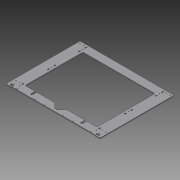
# Autodesk Inventor part: main_frame
Saved by Autodesk Inventor 2013 (Build 170138000, 138)
## iProperties
Created: 2013-11-17
Part Number: main_frame
Material: Generic
Document SubType Name: Modeling
Designer: Masta
Density: 1 g/cm^3
Author: Masta
Autodesk Inventor part; units mm, degrees
ref_plane "YZ Plane" through (0, 0, 0) normal (1, 0, 0) x (0, 1, 0)
ref_plane "XZ Plane" through (0, 0, 0) normal (0, 1, 0) x (-1, 0, 0)
ref_plane "XY Plane" through (0, 0, 0) normal (0, 0, 1) x (1, 0, 0)
sketch "Sketch1" plane through (0, 0, 0) normal (0, 0, 1) x (1, 0, 0)
  line L0 (36.0471, 18.5032) -> (31.0471, 23.3114)
  line L1 (31.0471, 383.5032) -> (36.0471, 388.5032)
  line L2 (36.0471, 388.5032) -> (396.0471, 388.5032)
  line L3 (396.0471, 388.5032) -> (401.0471, 383.5032)
  line L4 (401.0471, 23.5032) -> (396.0471, 18.5032)
  line L5 (376.0471, 18.5032) -> (374.0471, 20.5032)
  line L6 (374.0471, 20.5032) -> (58.0471, 20.5032)
  line L7 (58.0471, 20.5032) -> (56.0471, 18.5032)
  line L8 (111.0471, 58.5032) -> (91.0471, 58.5032)
  line L9 (91.0471, 58.5032) -> (86.0471, 63.5032)
  line L10 (86.0471, 63.5032) -> (86.0471, 343.5032)
  line L11 (86.0471, 343.5032) -> (91.0471, 348.5032)
  line L12 (91.0471, 348.5032) -> (341.0471, 348.5032)
  line L13 (341.0471, 348.5032) -> (346.0471, 343.5032)
  line L14 (346.0471, 343.5032) -> (346.0471, 63.5032)
  line L15 (346.0471, 63.5032) -> (341.0471, 58.5032)
  line L16 (341.0471, 58.5032) -> (321.0471, 58.5032)
  line L17 (211.0471, 33.5032) -> (221.0471, 33.5032)
  line L18 (221.0471, 33.5032) -> (246.0471, 58.5032)
  line L19 (211.0471, 33.5032) -> (186.0471, 58.5032)
  line L20 (141.0471, 58.5032) -> (186.0471, 58.5032)
  line L21 (246.0471, 58.5032) -> (291.0471, 58.5032)
  line L22 (381.0471, 24.5032) -> (381.3268, 24.54)
  line L23 (31.0471, 23.3114) -> (31.0471, 383.5032)
  line L24 (401.0471, 383.5032) -> (401.0471, 23.5032)
  line L25 (396.0471, 18.5032) -> (376.0471, 18.5032) construction
  line L26 (56.0471, 18.5032) -> (36.0471, 18.5032)
  line L27 (373.147, 30.54) -> (372.7474, 29.5753)
  line L28 (372.6111, 28.54) -> (372.7474, 27.5047)
  line L29 (375.5758, 32.4037) -> (374.6111, 32.0041)
  line L30 (385.6423, 32.4037) -> (384.6071, 32.54)
  line L31 (387.4355, 25.7116) -> (388.0712, 26.54)
  line L32 (386.6071, 25.0759) -> (387.4355, 25.7116)
  line L33 (385.6423, 24.6763) -> (386.6071, 25.0759)
  line L34 (374.6111, 25.0759) -> (375.5758, 24.6763)
  line L35 (375.5758, 24.6763) -> (376.6111, 24.54)
  line L36 (372.7474, 27.5047) -> (373.147, 26.54)
  line L37 (387.4355, 31.3684) -> (386.6071, 32.0041)
  line L38 (388.0712, 30.54) -> (387.4355, 31.3684)
  line L39 (376.6111, 32.54) -> (384.6071, 32.54)
  line L40 (374.6111, 32.0041) -> (373.7827, 31.3684)
  line L41 (373.7827, 31.3684) -> (373.147, 30.54)
  line L42 (373.7827, 25.7116) -> (374.6111, 25.0759)
  line L43 (388.4708, 29.5753) -> (388.0712, 30.54)
  line L44 (372.7474, 29.5753) -> (372.6111, 28.54)
  line L45 (373.147, 26.54) -> (373.7827, 25.7116)
  line L46 (388.4708, 27.5047) -> (388.6071, 28.54)
  line L47 (388.0712, 26.54) -> (388.4708, 27.5047)
  line L48 (376.6111, 32.54) -> (375.5758, 32.4037)
  line L49 (384.6739, 24.54) -> (385.6423, 24.6763)
  line L50 (376.6111, 24.54) -> (380.7674, 24.54)
  line L51 (388.6071, 28.54) -> (388.4708, 29.5753)
  line L52 (386.6071, 32.0041) -> (385.6423, 32.4037)
  line L53 (380.7674, 24.54) -> (381.0471, 24.5032)
  line L54 (380.7674, 24.54) -> (381.3268, 24.54)
  line L55 (381.3268, 24.54) -> (384.6739, 24.54)
  line L56 (43.0736, 28.54) -> (43.2099, 27.5047)
  line L57 (43.6095, 30.54) -> (43.2099, 29.5753)
  line L58 (46.0383, 32.4037) -> (45.0736, 32.0041)
  line L59 (56.1048, 32.4037) -> (55.0696, 32.54)
  line L60 (57.898, 25.7116) -> (58.5337, 26.54)
  line L61 (57.0696, 25.0759) -> (57.898, 25.7116)
  line L62 (56.1048, 24.6763) -> (57.0696, 25.0759)
  line L63 (45.0736, 25.0759) -> (46.0383, 24.6763)
  line L64 (46.0383, 24.6763) -> (47.0736, 24.54)
  line L65 (43.2099, 27.5047) -> (43.6095, 26.54)
  line L66 (57.898, 31.3684) -> (57.0696, 32.0041)
  line L67 (58.5337, 30.54) -> (57.898, 31.3684)
  line L68 (47.0736, 32.54) -> (55.0696, 32.54)
  line L69 (45.0736, 32.0041) -> (44.2452, 31.3684)
  line L70 (44.2452, 31.3684) -> (43.6095, 30.54)
  line L71 (44.2452, 25.7116) -> (45.0736, 25.0759)
  line L72 (58.9333, 29.5753) -> (58.5337, 30.54)
  line L73 (43.2099, 29.5753) -> (43.0736, 28.54)
  line L74 (43.6095, 26.54) -> (44.2452, 25.7116)
  line L75 (58.9333, 27.5047) -> (59.0696, 28.54)
  line L76 (58.5337, 26.54) -> (58.9333, 27.5047)
  line L77 (47.0736, 32.54) -> (46.0383, 32.4037)
  line L78 (55.1364, 24.54) -> (56.1048, 24.6763)
  line L79 (47.0736, 24.54) -> (55.1364, 24.54)
  line L80 (59.0696, 28.54) -> (58.9333, 29.5753)
  line L81 (57.0696, 32.0041) -> (56.1048, 32.4037)
  line L82 (354.7971, 370.2459) -> (354.7971, 379.2459)
  line L83 (354.7971, 379.2459) -> (361.2971, 379.2459)
  line L84 (361.2971, 379.2459) -> (361.2971, 370.2459)
  line L85 (361.2971, 370.2459) -> (354.7971, 370.2459)
  line L86 (354.7971, 337.9459) -> (354.7971, 346.9459)
  line L87 (354.7971, 346.9459) -> (361.2971, 346.9459)
  line L88 (361.2971, 346.9459) -> (361.2971, 337.9459)
  line L89 (361.2971, 337.9459) -> (354.7971, 337.9459)
  line L90 (354.7971, 215.1532) -> (354.7971, 224.1532)
  line L91 (354.7971, 224.1532) -> (361.2971, 224.1532)
  line L92 (361.2971, 224.1532) -> (361.2971, 215.1532)
  line L93 (361.2971, 215.1532) -> (354.7971, 215.1532)
  line L94 (354.7971, 182.8532) -> (354.7971, 191.8532)
  line L95 (354.7971, 191.8532) -> (361.2971, 191.8532)
  line L96 (361.2971, 191.8532) -> (361.2971, 182.8532)
  line L97 (361.2971, 182.8532) -> (354.7971, 182.8532)
  line L98 (354.7971, 55.1531) -> (354.7971, 64.1531)
  line L99 (354.7971, 64.1531) -> (361.2971, 64.1531)
  line L100 (361.2971, 64.1531) -> (361.2971, 55.1531)
  line L101 (361.2971, 55.1531) -> (354.7971, 55.1531)
  line L102 (70.7971, 370.2459) -> (70.7971, 379.2459)
  line L103 (70.7971, 379.2459) -> (77.2971, 379.2459)
  line L104 (77.2971, 379.2459) -> (77.2971, 370.2459)
  line L105 (77.2971, 370.2459) -> (70.7971, 370.2459)
  line L106 (70.7971, 337.9459) -> (70.7971, 346.9459)
  line L107 (70.7971, 346.9459) -> (77.2971, 346.9459)
  line L108 (77.2971, 346.9459) -> (77.2971, 337.9459)
  line L109 (77.2971, 337.9459) -> (70.7971, 337.9459)
  line L110 (70.7971, 215.1532) -> (70.7971, 224.1532)
  line L111 (70.7971, 224.1532) -> (77.2971, 224.1532)
  line L112 (77.2971, 224.1532) -> (77.2971, 215.1532)
  line L113 (77.2971, 215.1532) -> (70.7971, 215.1532)
  line L114 (70.7971, 182.8532) -> (70.7971, 191.8532)
  line L115 (70.7971, 191.8532) -> (77.2971, 191.8532)
  line L116 (77.2971, 191.8532) -> (77.2971, 182.8532)
  line L117 (77.2971, 182.8532) -> (70.7971, 182.8532)
  line L118 (70.7971, 55.1531) -> (70.7971, 64.1531)
  line L119 (70.7971, 64.1531) -> (77.2971, 64.1531)
  line L120 (77.2971, 64.1531) -> (77.2971, 55.1531)
  line L121 (77.2971, 55.1531) -> (70.7971, 55.1531)
  line L122 (359.8464, 203.5032) -> (359.785, 203.969)
  line L123 (359.785, 203.969) -> (359.6051, 204.4031)
  line L124 (359.6051, 204.4031) -> (359.319, 204.7759)
  line L125 (359.319, 204.7759) -> (358.9462, 205.0619)
  line L126 (358.9462, 205.0619) -> (358.512, 205.2416)
  line L127 (358.512, 205.2416) -> (358.0461, 205.3029)
  line L128 (358.0461, 205.3029) -> (357.5803, 205.2415)
  line L129 (357.5803, 205.2415) -> (357.1462, 205.0616)
  line L130 (357.1462, 205.0616) -> (356.7734, 204.7755)
  line L131 (356.7734, 204.7755) -> (356.4874, 204.4027)
  line L132 (356.4874, 204.4027) -> (356.3077, 203.9685)
  line L133 (356.3077, 203.9685) -> (356.2464, 203.5026)
  line L134 (356.2464, 203.5026) -> (356.3078, 203.0368)
  line L135 (356.3078, 203.0368) -> (356.4877, 202.6027)
  line L136 (356.4877, 202.6027) -> (356.7738, 202.2299)
  line L137 (356.7738, 202.2299) -> (357.1466, 201.9439)
  line L138 (357.1466, 201.9439) -> (357.5808, 201.7642)
  line L139 (357.5808, 201.7642) -> (358.0466, 201.7029)
  line L140 (358.0466, 201.7029) -> (358.5125, 201.7643)
  line L141 (358.5125, 201.7643) -> (358.9466, 201.9442)
  line L142 (358.9466, 201.9442) -> (359.3194, 202.2303)
  line L143 (359.3194, 202.2303) -> (359.6054, 202.6031)
  line L144 (359.6054, 202.6031) -> (359.7851, 203.0373)
  line L145 (359.7851, 203.0373) -> (359.8464, 203.5032)
  line L146 (359.8591, 358.5032) -> (359.7948, 358.9687)
  line L147 (359.7948, 358.9687) -> (359.6121, 359.4017)
  line L148 (359.6121, 359.4017) -> (359.3237, 359.7726)
  line L149 (359.3237, 359.7726) -> (358.949, 360.0562)
  line L150 (358.949, 360.0562) -> (358.5137, 360.2332)
  line L151 (358.5137, 360.2332) -> (358.0475, 360.2915)
  line L152 (358.0475, 360.2915) -> (357.582, 360.2272)
  line L153 (357.582, 360.2272) -> (357.1491, 360.0446)
  line L154 (357.1491, 360.0446) -> (356.7781, 359.7561)
  line L155 (356.7781, 359.7561) -> (356.4945, 359.3814)
  line L156 (356.4945, 359.3814) -> (356.3175, 358.9462)
  line L157 (356.3175, 358.9462) -> (356.2592, 358.4799)
  line L158 (356.2592, 358.4799) -> (356.3235, 358.0144)
  line L159 (356.3235, 358.0144) -> (356.5062, 357.5815)
  line L160 (356.5062, 357.5815) -> (356.7946, 357.2106)
  line L161 (356.7946, 357.2106) -> (357.1693, 356.9269)
  line L162 (357.1693, 356.9269) -> (357.6046, 356.7499)
  line L163 (357.6046, 356.7499) -> (358.0708, 356.6916)
  line L164 (358.0708, 356.6916) -> (358.5363, 356.756)
  line L165 (358.5363, 356.756) -> (358.9692, 356.9386)
  line L166 (358.9692, 356.9386) -> (359.3402, 357.2271)
  line L167 (359.3402, 357.2271) -> (359.6238, 357.6017)
  line L168 (359.6238, 357.6017) -> (359.8008, 358.037)
  line L169 (359.8008, 358.037) -> (359.8591, 358.5032)
  line L170 (371.0501, 380.2935) -> (370.5843, 380.2321)
  line L171 (372.8504, 378.4938) -> (372.789, 378.9596)
  line L172 (372.789, 378.9596) -> (372.6091, 379.3937)
  line L173 (372.6091, 379.3937) -> (372.323, 379.7665)
  line L174 (372.323, 379.7665) -> (371.9502, 380.0525)
  line L175 (370.5843, 380.2321) -> (370.1502, 380.0522)
  line L176 (370.1502, 380.0522) -> (369.7774, 379.7661)
  line L177 (369.7774, 379.7661) -> (369.4914, 379.3933)
  line L178 (371.0506, 376.6935) -> (371.5165, 376.7549)
  line L179 (371.5165, 376.7549) -> (371.9506, 376.9348)
  line L180 (371.9502, 380.0525) -> (371.516, 380.2322)
  line L181 (371.516, 380.2322) -> (371.0501, 380.2935)
  line L182 (369.4914, 379.3933) -> (369.3116, 378.9591)
  line L183 (369.3116, 378.9591) -> (369.2504, 378.4933)
  line L184 (369.2504, 378.4933) -> (369.3118, 378.0274)
  line L185 (369.3118, 378.0274) -> (369.4917, 377.5933)
  line L186 (371.9506, 376.9348) -> (372.3234, 377.2209)
  line L187 (372.3234, 377.2209) -> (372.6094, 377.5937)
  line L188 (372.6094, 377.5937) -> (372.7891, 378.0279)
  line L189 (372.7891, 378.0279) -> (372.8504, 378.4938)
  line L190 (369.4917, 377.5933) -> (369.7778, 377.2205)
  line L191 (369.7778, 377.2205) -> (370.1506, 376.9345)
  line L192 (370.1506, 376.9345) -> (370.5848, 376.7548)
  line L193 (370.5848, 376.7548) -> (371.0506, 376.6935)
  line L194 (392.7633, 378.9927) -> (392.5834, 379.4268)
  line L195 (390.1245, 380.0852) -> (389.7517, 379.7991)
  line L196 (389.7517, 379.7991) -> (389.4657, 379.4263)
  line L197 (389.7521, 377.2536) -> (390.1249, 376.9676)
  line L198 (390.1249, 376.9676) -> (390.5591, 376.7878)
  line L199 (390.5591, 376.7878) -> (391.025, 376.7265)
  line L200 (389.2861, 378.0604) -> (389.466, 377.6263)
  line L201 (389.466, 377.6263) -> (389.7521, 377.2536)
  line L202 (389.4657, 379.4263) -> (389.286, 378.9922)
  line L203 (389.286, 378.9922) -> (389.2247, 378.5263)
  line L204 (389.2247, 378.5263) -> (389.2861, 378.0604)
  line L205 (391.9245, 380.0855) -> (391.4903, 380.2653)
  line L206 (392.2973, 379.7995) -> (391.9245, 380.0855)
  line L207 (392.5834, 379.4268) -> (392.2973, 379.7995)
  line L208 (391.4903, 380.2653) -> (391.0244, 380.3265)
  line L209 (391.0244, 380.3265) -> (390.5586, 380.2651)
  line L210 (390.5586, 380.2651) -> (390.1245, 380.0852)
  line L211 (392.8247, 378.5268) -> (392.7633, 378.9927)
  line L212 (392.7634, 378.0609) -> (392.8247, 378.5268)
  line L213 (391.025, 376.7265) -> (391.4908, 376.7879)
  line L214 (391.4908, 376.7879) -> (391.9249, 376.9678)
  line L215 (391.9249, 376.9678) -> (392.2977, 377.2539)
  line L216 (392.2977, 377.2539) -> (392.5837, 377.6268)
  line L217 (392.5837, 377.6268) -> (392.7634, 378.0609)
  line L218 (370.5952, 60.2328) -> (370.1611, 60.0529)
  line L219 (372.62, 59.3944) -> (372.3339, 59.7672)
  line L220 (369.3226, 58.9598) -> (369.2613, 58.494)
  line L221 (372.7999, 58.9603) -> (372.62, 59.3944)
  line L222 (369.7883, 59.7668) -> (369.5023, 59.394)
  line L223 (372.8613, 58.4945) -> (372.7999, 58.9603)
  line L224 (370.1611, 60.0529) -> (369.7883, 59.7668)
  line L225 (371.5269, 60.2329) -> (371.0611, 60.2942)
  line L226 (370.1615, 56.9352) -> (370.5957, 56.7555)
  line L227 (371.5274, 56.7556) -> (371.9615, 56.9355)
  line L228 (371.9615, 56.9355) -> (372.3343, 57.2216)
  line L229 (369.5026, 57.594) -> (369.7887, 57.2212)
  line L230 (369.7887, 57.2212) -> (370.1615, 56.9352)
  line L231 (371.0611, 60.2942) -> (370.5952, 60.2328)
  line L232 (370.5957, 56.7555) -> (371.0616, 56.6942)
  line L233 (371.0616, 56.6942) -> (371.5274, 56.7556)
  line L234 (372.3339, 59.7672) -> (371.9611, 60.0532)
  line L235 (371.9611, 60.0532) -> (371.5269, 60.2329)
  line L236 (372.6203, 57.5944) -> (372.8, 58.0286)
  line L237 (372.8, 58.0286) -> (372.8613, 58.4945)
  line L238 (369.2613, 58.494) -> (369.3227, 58.0281)
  line L239 (369.3227, 58.0281) -> (369.5026, 57.594)
  line L240 (372.3343, 57.2216) -> (372.6203, 57.5944)
  line L241 (369.5023, 59.394) -> (369.3226, 58.9598)
  line L242 (391.5063, 56.7108) -> (391.9404, 56.8907)
  line L243 (391.9404, 56.8907) -> (392.3131, 57.1768)
  line L244 (392.3131, 57.1768) -> (392.5991, 57.5496)
  line L245 (390.574, 60.188) -> (390.1399, 60.0081)
  line L246 (390.1399, 60.0081) -> (389.7672, 59.722)
  line L247 (389.4814, 57.5492) -> (389.7675, 57.1764)
  line L248 (389.7675, 57.1764) -> (390.1404, 56.8904)
  line L249 (389.2402, 58.4492) -> (389.3016, 57.9833)
  line L250 (389.3016, 57.9833) -> (389.4814, 57.5492)
  line L251 (389.7672, 59.722) -> (389.4812, 59.3492)
  line L252 (389.4812, 59.3492) -> (389.3014, 58.915)
  line L253 (389.3014, 58.915) -> (389.2402, 58.4492)
  line L254 (390.1404, 56.8904) -> (390.5745, 56.7107)
  line L255 (390.5745, 56.7107) -> (391.0404, 56.6494)
  line L256 (391.0404, 56.6494) -> (391.5063, 56.7108)
  line L257 (391.5058, 60.1882) -> (391.0399, 60.2494)
  line L258 (392.5989, 59.3496) -> (392.3128, 59.7224)
  line L259 (392.7788, 58.9155) -> (392.5989, 59.3496)
  line L260 (392.3128, 59.7224) -> (391.9399, 60.0084)
  line L261 (391.9399, 60.0084) -> (391.5058, 60.1882)
  line L262 (392.8402, 58.4497) -> (392.7788, 58.9155)
  line L263 (391.0399, 60.2494) -> (390.574, 60.188)
  line L264 (392.5991, 57.5496) -> (392.7789, 57.9838)
  line L265 (392.7789, 57.9838) -> (392.8402, 58.4497)
  line L266 (382.6094, 39.3708) -> (382.3233, 39.7435)
  line L267 (382.7895, 38.0049) -> (382.8507, 38.4708)
  line L268 (379.7778, 39.7432) -> (379.4918, 39.3704)
  line L269 (379.4918, 39.3704) -> (379.312, 38.9362)
  line L270 (379.312, 38.9362) -> (379.2507, 38.4703)
  line L271 (379.7781, 37.1976) -> (380.151, 36.9116)
  line L272 (380.151, 36.9116) -> (380.5851, 36.7318)
  line L273 (380.5851, 36.7318) -> (381.051, 36.6706)
  line L274 (381.051, 36.6706) -> (381.5169, 36.732)
  line L275 (381.5169, 36.732) -> (381.951, 36.9119)
  line L276 (381.951, 36.9119) -> (382.3237, 37.198)
  line L277 (382.3237, 37.198) -> (382.6097, 37.5708)
  line L278 (382.6097, 37.5708) -> (382.7895, 38.0049)
  line L279 (381.0505, 40.2706) -> (380.5846, 40.2092)
  line L280 (380.5846, 40.2092) -> (380.1505, 40.0293)
  line L281 (380.1505, 40.0293) -> (379.7778, 39.7432)
  line L282 (379.2507, 38.4703) -> (379.3121, 38.0045)
  line L283 (379.3121, 38.0045) -> (379.492, 37.5704)
  line L284 (379.492, 37.5704) -> (379.7781, 37.1976)
  line L285 (382.8507, 38.4708) -> (382.7893, 38.9367)
  line L286 (382.7893, 38.9367) -> (382.6094, 39.3708)
  line L287 (382.3233, 39.7435) -> (381.9505, 40.0295)
  line L288 (381.9505, 40.0295) -> (381.5164, 40.2093)
  line L289 (381.5164, 40.2093) -> (381.0505, 40.2706)
  line L290 (359.8464, 43.5032) -> (359.7851, 43.9689)
  line L291 (359.7851, 43.9689) -> (359.6053, 44.4028)
  line L292 (359.6053, 44.4028) -> (359.3194, 44.7755)
  line L293 (359.3194, 44.7755) -> (358.9467, 45.0614)
  line L294 (358.9467, 45.0614) -> (358.5128, 45.2411)
  line L295 (358.5128, 45.2411) -> (358.0471, 45.3025)
  line L296 (358.0471, 45.3025) -> (357.5814, 45.2411)
  line L297 (357.5814, 45.2411) -> (357.1475, 45.0614)
  line L298 (357.1475, 45.0614) -> (356.7748, 44.7755)
  line L299 (356.7748, 44.7755) -> (356.4889, 44.4028)
  line L300 (356.4889, 44.4028) -> (356.3091, 43.9689)
  line L301 (356.3091, 43.9689) -> (356.2478, 43.5032)
  line L302 (356.2478, 43.5032) -> (356.3091, 43.0375)
  line L303 (356.3091, 43.0375) -> (356.4889, 42.6035)
  line L304 (356.4889, 42.6035) -> (356.7748, 42.2309)
  line L305 (356.7748, 42.2309) -> (357.1475, 41.945)
  line L306 (357.1475, 41.945) -> (357.5814, 41.7652)
  line L307 (357.5814, 41.7652) -> (358.0471, 41.7039)
  line L308 (358.0471, 41.7039) -> (358.5128, 41.7652)
  line L309 (358.5128, 41.7652) -> (358.9467, 41.945)
  line L310 (358.9467, 41.945) -> (359.3194, 42.2309)
  line L311 (359.3194, 42.2309) -> (359.6053, 42.6035)
  line L312 (359.6053, 42.6035) -> (359.7851, 43.0375)
  line L313 (359.7851, 43.0375) -> (359.8464, 43.5032)
  line L314 (41.4817, 60.2626) -> (41.0158, 60.3239)
  line L315 (41.0158, 60.3239) -> (40.5499, 60.2625)
  line L316 (40.5499, 60.2625) -> (40.1158, 60.0826)
  line L317 (40.1158, 60.0826) -> (39.7431, 59.7965)
  line L318 (39.7431, 59.7965) -> (39.4571, 59.4236)
  line L319 (39.4571, 59.4236) -> (39.2773, 58.9895)
  line L320 (42.289, 57.2513) -> (42.575, 57.6241)
  line L321 (42.575, 57.6241) -> (42.7548, 58.0582)
  line L322 (42.7548, 58.0582) -> (42.816, 58.5241)
  line L323 (39.2773, 58.9895) -> (39.216, 58.5236)
  line L324 (39.216, 58.5236) -> (39.2774, 58.0577)
  line L325 (39.2774, 58.0577) -> (39.4573, 57.6236)
  line L326 (42.7546, 58.99) -> (42.5747, 59.4241)
  line L327 (42.816, 58.5241) -> (42.7546, 58.99)
  line L328 (39.4573, 57.6236) -> (39.7434, 57.2509)
  line L329 (39.7434, 57.2509) -> (40.1163, 56.9649)
  line L330 (40.1163, 56.9649) -> (40.5504, 56.7851)
  line L331 (40.5504, 56.7851) -> (41.0163, 56.7239)
  line L332 (41.0163, 56.7239) -> (41.4822, 56.7853)
  line L333 (41.4822, 56.7853) -> (41.9163, 56.9651)
  line L334 (41.9163, 56.9651) -> (42.289, 57.2513)
  line L335 (41.9158, 60.0828) -> (41.4817, 60.2626)
  line L336 (42.2886, 59.7968) -> (41.9158, 60.0828)
  line L337 (42.5747, 59.4241) -> (42.2886, 59.7968)
  line L338 (60.5638, 60.2625) -> (60.1297, 60.0826)
  line L339 (60.1297, 60.0826) -> (59.7569, 59.7965)
  line L340 (59.7569, 59.7965) -> (59.4709, 59.4236)
  line L341 (62.8299, 58.5241) -> (62.7685, 58.99)
  line L342 (62.7685, 58.99) -> (62.5886, 59.4241)
  line L343 (62.5886, 59.4241) -> (62.3025, 59.7968)
  line L344 (61.4955, 60.2626) -> (61.0296, 60.3239)
  line L345 (61.0296, 60.3239) -> (60.5638, 60.2625)
  line L346 (59.7573, 57.2509) -> (60.1301, 56.9649)
  line L347 (60.1301, 56.9649) -> (60.5642, 56.7851)
  line L348 (60.5642, 56.7851) -> (61.0301, 56.7239)
  line L349 (61.0301, 56.7239) -> (61.496, 56.7853)
  line L350 (61.496, 56.7853) -> (61.9301, 56.9651)
  line L351 (61.9301, 56.9651) -> (62.3028, 57.2513)
  line L352 (62.3025, 59.7968) -> (61.9296, 60.0828)
  line L353 (61.9296, 60.0828) -> (61.4955, 60.2626)
  line L354 (59.4709, 59.4236) -> (59.2911, 58.9895)
  line L355 (59.2911, 58.9895) -> (59.2299, 58.5236)
  line L356 (59.2299, 58.5236) -> (59.2913, 58.0577)
  line L357 (59.2913, 58.0577) -> (59.4712, 57.6236)
  line L358 (59.4712, 57.6236) -> (59.7573, 57.2509)
  line L359 (62.3028, 57.2513) -> (62.5888, 57.6241)
  line L360 (62.5888, 57.6241) -> (62.7686, 58.0582)
  line L361 (62.7686, 58.0582) -> (62.8299, 58.5241)
  line L362 (52.5817, 39.4102) -> (52.2956, 39.783)
  line L363 (52.7616, 38.9761) -> (52.5817, 39.4102)
  line L364 (52.823, 38.5103) -> (52.7616, 38.9761)
  line L365 (52.2956, 39.783) -> (51.9227, 40.069)
  line L366 (49.464, 39.4098) -> (49.2842, 38.9756)
  line L367 (49.2842, 38.9756) -> (49.223, 38.5098)
  line L368 (49.223, 38.5098) -> (49.2844, 38.0439)
  line L369 (49.2844, 38.0439) -> (49.4642, 37.6098)
  line L370 (49.4642, 37.6098) -> (49.7503, 37.237)
  line L371 (49.7503, 37.237) -> (50.1232, 36.951)
  line L372 (50.1232, 36.951) -> (50.5573, 36.7713)
  line L373 (50.5573, 36.7713) -> (51.0232, 36.71)
  line L374 (51.0232, 36.71) -> (51.4891, 36.7714)
  line L375 (51.4891, 36.7714) -> (51.9232, 36.9513)
  line L376 (51.9232, 36.9513) -> (52.2959, 37.2374)
  line L377 (52.2959, 37.2374) -> (52.5819, 37.6102)
  line L378 (52.5819, 37.6102) -> (52.7617, 38.0444)
  line L379 (52.7617, 38.0444) -> (52.823, 38.5103)
  line L380 (51.9227, 40.069) -> (51.4886, 40.2488)
  line L381 (51.4886, 40.2488) -> (51.0227, 40.31)
  line L382 (51.0227, 40.31) -> (50.5568, 40.2486)
  line L383 (50.5568, 40.2486) -> (50.1227, 40.0687)
  line L384 (50.1227, 40.0687) -> (49.75, 39.7826)
  line L385 (49.75, 39.7826) -> (49.464, 39.4098)
  line L386 (72.7577, 42.2405) -> (73.1305, 41.9545)
  line L387 (73.1305, 41.9545) -> (73.5647, 41.7748)
  line L388 (73.5647, 41.7748) -> (74.0306, 41.7135)
  line L389 (74.0306, 41.7135) -> (74.4964, 41.7749)
  line L390 (74.4964, 41.7749) -> (74.9305, 41.9548)
  line L391 (75.7689, 43.9796) -> (75.589, 44.4137)
  line L392 (74.9301, 45.0725) -> (74.4959, 45.2522)
  line L393 (74.4959, 45.2522) -> (74.0301, 45.3135)
  line L394 (74.0301, 45.3135) -> (73.5642, 45.2521)
  line L395 (73.5642, 45.2521) -> (73.1301, 45.0722)
  line L396 (73.1301, 45.0722) -> (72.7573, 44.7861)
  line L397 (75.8303, 43.5137) -> (75.7689, 43.9796)
  line L398 (74.9305, 41.9548) -> (75.3033, 42.2409)
  line L399 (75.3033, 42.2409) -> (75.5893, 42.6137)
  line L400 (75.5893, 42.6137) -> (75.7691, 43.0479)
  line L401 (75.7691, 43.0479) -> (75.8303, 43.5137)
  line L402 (72.7573, 44.7861) -> (72.4713, 44.4133)
  line L403 (72.4713, 44.4133) -> (72.2916, 43.9791)
  line L404 (72.2916, 43.9791) -> (72.2303, 43.5132)
  line L405 (72.2303, 43.5132) -> (72.2917, 43.0474)
  line L406 (72.2917, 43.0474) -> (72.4716, 42.6133)
  line L407 (72.4716, 42.6133) -> (72.7577, 42.2405)
  line L408 (75.589, 44.4137) -> (75.3029, 44.7865)
  line L409 (75.3029, 44.7865) -> (74.9301, 45.0725)
  line L410 (73.6067, 201.7613) -> (74.0726, 201.7)
  line L411 (74.0726, 201.7) -> (74.5385, 201.7614)
  line L412 (74.5385, 201.7614) -> (74.9726, 201.9413)
  line L413 (74.0721, 205.3) -> (73.6062, 205.2386)
  line L414 (73.6062, 205.2386) -> (73.1721, 205.0588)
  line L415 (73.1721, 205.0588) -> (72.7994, 204.7726)
  line L416 (75.811, 203.9662) -> (75.6311, 204.4003)
  line L417 (72.5134, 204.3998) -> (72.3336, 203.9657)
  line L418 (72.3336, 203.9657) -> (72.2724, 203.4998)
  line L419 (74.9726, 201.9413) -> (75.3453, 202.2274)
  line L420 (75.3453, 202.2274) -> (75.6313, 202.6003)
  line L421 (72.3338, 203.0339) -> (72.5137, 202.5998)
  line L422 (72.5137, 202.5998) -> (72.7998, 202.2271)
  line L423 (72.2724, 203.4998) -> (72.3338, 203.0339)
  line L424 (74.9721, 205.059) -> (74.538, 205.2388)
  line L425 (72.7994, 204.7726) -> (72.5134, 204.3998)
  line L426 (75.345, 204.773) -> (74.9721, 205.059)
  line L427 (75.6311, 204.4003) -> (75.345, 204.773)
  line L428 (74.538, 205.2388) -> (74.0721, 205.3)
  line L429 (75.8724, 203.5003) -> (75.811, 203.9662)
  line L430 (72.7998, 202.2271) -> (73.1726, 201.9411)
  line L431 (73.1726, 201.9411) -> (73.6067, 201.7613)
  line L432 (75.6313, 202.6003) -> (75.8111, 203.0344)
  line L433 (75.8111, 203.0344) -> (75.8724, 203.5003)
  line L434 (41.0518, 376.7166) -> (41.5177, 376.778)
  line L435 (41.5177, 376.778) -> (41.9518, 376.9579)
  line L436 (41.9518, 376.9579) -> (42.3246, 377.244)
  line L437 (42.3246, 377.244) -> (42.6106, 377.6169)
  line L438 (39.3129, 378.9823) -> (39.2516, 378.5164)
  line L439 (39.2516, 378.5164) -> (39.313, 378.0505)
  line L440 (40.1514, 380.0753) -> (39.7786, 379.7892)
  line L441 (41.5172, 380.2554) -> (41.0513, 380.3166)
  line L442 (41.9514, 380.0756) -> (41.5172, 380.2554)
  line L443 (42.6106, 377.6169) -> (42.7903, 378.051)
  line L444 (42.7903, 378.051) -> (42.8516, 378.5169)
  line L445 (39.313, 378.0505) -> (39.4929, 377.6164)
  line L446 (39.4929, 377.6164) -> (39.779, 377.2437)
  line L447 (41.0513, 380.3166) -> (40.5855, 380.2552)
  line L448 (40.5855, 380.2552) -> (40.1514, 380.0753)
  line L449 (39.7786, 379.7892) -> (39.4926, 379.4164)
  line L450 (39.4926, 379.4164) -> (39.3129, 378.9823)
  line L451 (42.3242, 379.7896) -> (41.9514, 380.0756)
  line L452 (42.6103, 379.4169) -> (42.3242, 379.7896)
  line L453 (42.7902, 378.9828) -> (42.6103, 379.4169)
  line L454 (42.8516, 378.5169) -> (42.7902, 378.9828)
  line L455 (39.779, 377.2437) -> (40.1518, 376.9577)
  line L456 (40.1518, 376.9577) -> (40.586, 376.7779)
  line L457 (40.586, 376.7779) -> (41.0518, 376.7166)
  line L458 (59.7971, 379.7892) -> (59.5111, 379.4164)
  line L459 (59.5111, 379.4164) -> (59.3313, 378.9823)
  line L460 (59.3313, 378.9823) -> (59.27, 378.5164)
  line L461 (59.27, 378.5164) -> (59.3314, 378.0505)
  line L462 (59.3314, 378.0505) -> (59.5113, 377.6164)
  line L463 (61.5357, 380.2554) -> (61.0698, 380.3166)
  line L464 (61.9703, 376.9579) -> (62.343, 377.244)
  line L465 (62.343, 377.244) -> (62.629, 377.6169)
  line L466 (62.629, 377.6169) -> (62.8088, 378.051)
  line L467 (62.8088, 378.051) -> (62.87, 378.5169)
  line L468 (61.9698, 380.0756) -> (61.5357, 380.2554)
  line L469 (61.0698, 380.3166) -> (60.6039, 380.2552)
  line L470 (62.87, 378.5169) -> (62.8086, 378.9828)
  line L471 (62.8086, 378.9828) -> (62.6287, 379.4169)
  line L472 (62.6287, 379.4169) -> (62.3426, 379.7896)
  line L473 (62.3426, 379.7896) -> (61.9698, 380.0756)
  line L474 (59.5113, 377.6164) -> (59.7974, 377.2437)
  line L475 (59.7974, 377.2437) -> (60.1703, 376.9577)
  line L476 (60.1703, 376.9577) -> (60.6044, 376.7779)
  line L477 (60.6044, 376.7779) -> (61.0703, 376.7166)
  line L478 (61.0703, 376.7166) -> (61.5362, 376.778)
  line L479 (61.5362, 376.778) -> (61.9703, 376.9579)
  line L480 (60.6039, 380.2552) -> (60.1698, 380.0753)
  line L481 (60.1698, 380.0753) -> (59.7971, 379.7892)
  line L482 (75.345, 359.7712) -> (74.9721, 360.0572)
  line L483 (72.5137, 357.598) -> (72.7998, 357.2252)
  line L484 (72.7998, 357.2252) -> (73.1726, 356.9392)
  line L485 (73.1726, 356.9392) -> (73.6067, 356.7595)
  line L486 (73.6067, 356.7595) -> (74.0726, 356.6982)
  line L487 (74.0726, 356.6982) -> (74.5385, 356.7596)
  line L488 (74.538, 360.2369) -> (74.0721, 360.2982)
  line L489 (74.0721, 360.2982) -> (73.6062, 360.2368)
  line L490 (73.6062, 360.2368) -> (73.1721, 360.0569)
  line L491 (73.1721, 360.0569) -> (72.7994, 359.7708)
  line L492 (72.7994, 359.7708) -> (72.5134, 359.398)
  line L493 (72.5134, 359.398) -> (72.3336, 358.9638)
  line L494 (72.3336, 358.9638) -> (72.2724, 358.4979)
  line L495 (72.2724, 358.4979) -> (72.3338, 358.0321)
  line L496 (72.3338, 358.0321) -> (72.5137, 357.598)
  line L497 (75.6311, 359.3984) -> (75.345, 359.7712)
  line L498 (75.811, 358.9643) -> (75.6311, 359.3984)
  line L499 (75.8724, 358.4984) -> (75.811, 358.9643)
  line L500 (74.5385, 356.7596) -> (74.9726, 356.9395)
  line L501 (74.9726, 356.9395) -> (75.3453, 357.2256)
  line L502 (75.3453, 357.2256) -> (75.6313, 357.5984)
  line L503 (75.6313, 357.5984) -> (75.8111, 358.0326)
  line L504 (75.8111, 358.0326) -> (75.8724, 358.4984)
  line L505 (74.9721, 360.0572) -> (74.538, 360.2369)
  line L506 (82.8471, 24.5032) -> (82.7858, 24.9691)
  line L507 (82.7858, 24.9691) -> (82.606, 25.4032)
  line L508 (82.606, 25.4032) -> (82.3199, 25.776)
  line L509 (82.3199, 25.776) -> (81.9471, 26.062)
  line L510 (81.9471, 26.062) -> (81.513, 26.2418)
  line L511 (81.513, 26.2418) -> (81.0471, 26.3032)
  line L512 (81.0471, 26.3032) -> (80.5813, 26.2418)
  line L513 (80.5813, 26.2418) -> (80.1471, 26.062)
  line L514 (80.1471, 26.062) -> (79.7743, 25.776)
  line L515 (79.7743, 25.776) -> (79.4883, 25.4032)
  line L516 (79.4883, 25.4032) -> (79.3085, 24.9691)
  line L517 (79.3085, 24.9691) -> (79.2471, 24.5032)
  line L518 (79.2471, 24.5032) -> (79.3085, 24.0373)
  line L519 (79.3085, 24.0373) -> (79.4883, 23.6032)
  line L520 (79.4883, 23.6032) -> (79.7743, 23.2304)
  line L521 (79.7743, 23.2304) -> (80.1471, 22.9443)
  line L522 (80.1471, 22.9443) -> (80.5813, 22.7645)
  line L523 (80.5813, 22.7645) -> (81.0471, 22.7032)
  line L524 (81.0471, 22.7032) -> (81.513, 22.7645)
  line L525 (81.513, 22.7645) -> (81.9471, 22.9443)
  line L526 (81.9471, 22.9443) -> (82.3199, 23.2304)
  line L527 (82.3199, 23.2304) -> (82.606, 23.6032)
  line L528 (82.606, 23.6032) -> (82.7858, 24.0373)
  line L529 (82.7858, 24.0373) -> (82.8471, 24.5032)
  line L530 (172.8471, 24.5032) -> (172.7858, 24.9691)
  line L531 (172.7858, 24.9691) -> (172.606, 25.4032)
  line L532 (172.606, 25.4032) -> (172.3199, 25.776)
  line L533 (172.3199, 25.776) -> (171.9471, 26.062)
  line L534 (171.9471, 26.062) -> (171.513, 26.2418)
  line L535 (171.513, 26.2418) -> (171.0471, 26.3032)
  line L536 (171.0471, 26.3032) -> (170.5813, 26.2418)
  line L537 (170.5813, 26.2418) -> (170.1471, 26.062)
  line L538 (170.1471, 26.062) -> (169.7743, 25.776)
  line L539 (169.7743, 25.776) -> (169.4883, 25.4032)
  line L540 (169.4883, 25.4032) -> (169.3085, 24.9691)
  line L541 (169.3085, 24.9691) -> (169.2471, 24.5032)
  line L542 (169.2471, 24.5032) -> (169.3085, 24.0373)
  line L543 (169.3085, 24.0373) -> (169.4883, 23.6032)
  line L544 (169.4883, 23.6032) -> (169.7743, 23.2304)
  line L545 (169.7743, 23.2304) -> (170.1471, 22.9443)
  line L546 (170.1471, 22.9443) -> (170.5813, 22.7645)
  line L547 (170.5813, 22.7645) -> (171.0471, 22.7032)
  line L548 (171.0471, 22.7032) -> (171.513, 22.7645)
  line L549 (171.513, 22.7645) -> (171.9471, 22.9443)
  line L550 (171.9471, 22.9443) -> (172.3199, 23.2304)
  line L551 (172.3199, 23.2304) -> (172.606, 23.6032)
  line L552 (172.606, 23.6032) -> (172.7858, 24.0373)
  line L553 (172.7858, 24.0373) -> (172.8471, 24.5032)
  line L554 (262.8471, 24.5032) -> (262.7858, 24.9691)
  line L555 (262.7858, 24.9691) -> (262.606, 25.4032)
  line L556 (262.606, 25.4032) -> (262.3199, 25.776)
  line L557 (262.3199, 25.776) -> (261.9471, 26.062)
  line L558 (261.9471, 26.062) -> (261.513, 26.2418)
  line L559 (261.513, 26.2418) -> (261.0471, 26.3032)
  line L560 (261.0471, 26.3032) -> (260.5812, 26.2418)
  line L561 (260.5812, 26.2418) -> (260.1471, 26.062)
  line L562 (260.1471, 26.062) -> (259.7743, 25.776)
  line L563 (259.7743, 25.776) -> (259.4883, 25.4032)
  line L564 (259.4883, 25.4032) -> (259.3085, 24.9691)
  line L565 (259.3085, 24.9691) -> (259.2471, 24.5032)
  line L566 (259.2471, 24.5032) -> (259.3085, 24.0373)
  line L567 (259.3085, 24.0373) -> (259.4883, 23.6032)
  line L568 (259.4883, 23.6032) -> (259.7743, 23.2304)
  line L569 (259.7743, 23.2304) -> (260.1471, 22.9443)
  line L570 (260.1471, 22.9443) -> (260.5812, 22.7645)
  line L571 (260.5812, 22.7645) -> (261.0471, 22.7032)
  line L572 (261.0471, 22.7032) -> (261.513, 22.7645)
  line L573 (261.513, 22.7645) -> (261.9471, 22.9443)
  line L574 (261.9471, 22.9443) -> (262.3199, 23.2304)
  line L575 (262.3199, 23.2304) -> (262.606, 23.6032)
  line L576 (262.606, 23.6032) -> (262.7858, 24.0373)
  line L577 (262.7858, 24.0373) -> (262.8471, 24.5032)
  line L578 (349.2471, 24.5032) -> (349.3084, 24.0373)
  line L579 (349.3084, 24.0373) -> (349.4883, 23.6032)
  line L580 (349.4883, 23.6032) -> (349.7743, 23.2304)
  line L581 (349.7743, 23.2304) -> (350.1471, 22.9443)
  line L582 (350.1471, 22.9443) -> (350.5812, 22.7645)
  line L583 (350.5812, 22.7645) -> (351.0471, 22.7032)
  line L584 (351.0471, 22.7032) -> (351.513, 22.7645)
  line L585 (351.513, 22.7645) -> (351.9471, 22.9443)
  line L586 (351.9471, 22.9443) -> (352.3199, 23.2304)
  line L587 (352.3199, 23.2304) -> (352.606, 23.6032)
  line L588 (352.606, 23.6032) -> (352.7858, 24.0373)
  line L589 (352.7858, 24.0373) -> (352.8471, 24.5032)
  line L590 (352.8471, 24.5032) -> (352.7858, 24.9691)
  line L591 (352.7858, 24.9691) -> (352.606, 25.4032)
  line L592 (352.606, 25.4032) -> (352.3199, 25.776)
  line L593 (352.3199, 25.776) -> (351.9471, 26.062)
  line L594 (351.9471, 26.062) -> (351.513, 26.2418)
  line L595 (351.513, 26.2418) -> (351.0471, 26.3032)
  line L596 (351.0471, 26.3032) -> (350.5812, 26.2418)
  line L597 (350.5812, 26.2418) -> (350.1471, 26.062)
  line L598 (350.1471, 26.062) -> (349.7743, 25.776)
  line L599 (349.7743, 25.776) -> (349.4883, 25.4032)
  line L600 (349.4883, 25.4032) -> (349.3084, 24.9691)
  line L601 (349.3084, 24.9691) -> (349.2471, 24.5032)
  line L602 (126.0471, 52.5032) -> (126.0471, 38.4376)
  line L603 (126.0471, 38.4376) -> (126.2092, 37.2069)
  line L604 (126.2092, 37.2069) -> (126.7095, 35.9989)
  line L605 (126.7095, 35.9989) -> (127.5055, 34.9615)
  line L606 (127.5055, 34.9615) -> (128.5428, 34.1656)
  line L607 (128.5428, 34.1656) -> (129.7508, 33.6652)
  line L608 (129.7508, 33.6652) -> (131.0471, 33.4946)
  line L609 (131.0471, 33.4946) -> (132.3435, 33.6652)
  line L610 (132.3435, 33.6652) -> (133.5514, 34.1656)
  line L611 (133.5514, 34.1656) -> (134.5888, 34.9615)
  line L612 (134.5888, 34.9615) -> (135.3847, 35.9989)
  line L613 (135.3847, 35.9989) -> (135.8851, 37.2069)
  line L614 (135.8851, 37.2069) -> (136.0471, 38.4376)
  line L615 (136.0471, 38.4376) -> (136.0471, 52.5032)
  line L616 (126.0471, 52.5032) -> (126.0471, 53.5032)
  line L617 (136.0471, 53.5032) -> (141.0471, 58.5032)
  line L618 (136.0471, 52.5032) -> (136.0471, 53.5032)
  line L619 (296.0471, 52.5032) -> (296.0471, 38.4376)
  line L620 (296.0471, 38.4376) -> (296.2092, 37.2069)
  line L621 (296.2092, 37.2069) -> (296.7095, 35.9989)
  line L622 (296.7095, 35.9989) -> (297.5055, 34.9615)
  line L623 (297.5055, 34.9615) -> (298.5428, 34.1656)
  line L624 (298.5428, 34.1656) -> (299.7508, 33.6652)
  line L625 (299.7508, 33.6652) -> (301.0471, 33.4946)
  line L626 (301.0471, 33.4946) -> (302.3434, 33.6652)
  line L627 (302.3434, 33.6652) -> (303.5514, 34.1656)
  line L628 (303.5514, 34.1656) -> (304.5887, 34.9615)
  line L629 (304.5887, 34.9615) -> (305.3847, 35.9989)
  line L630 (305.3847, 35.9989) -> (305.8851, 37.2069)
  line L631 (305.8851, 37.2069) -> (306.0471, 38.4376)
  line L632 (306.0471, 38.4376) -> (306.0471, 52.5032)
  line L633 (296.0471, 53.5032) -> (291.0471, 58.5032)
  line L634 (296.0471, 52.5032) -> (296.0471, 53.5032)
  line L635 (306.0471, 52.5032) -> (306.0471, 53.5032)
  line L636 (111.0471, 58.5032) -> (121.0471, 58.5032)
  line L637 (121.0471, 58.5032) -> (126.0471, 53.5032)
  line L638 (321.0471, 58.5032) -> (311.0471, 58.5032)
  line L639 (306.0471, 53.5032) -> (311.0471, 58.5032)
  line L640 (967.1745, 43.6282) -> (967.1745, 413.6282)
  line L641 (967.1745, 413.6282) -> (497.1745, 413.6282)
  line L642 (497.1745, 413.6282) -> (497.1745, 43.6282)
  circle A0 centre (957.1745, 403.6282) radius 1.8
  circle A1 centre (937.1745, 403.6282) radius 1.8
  circle A2 centre (957.1745, 83.6282) radius 1.8
  circle A3 centre (937.1745, 83.6282) radius 1.8
  line L643 (732.1745, 413.6282) -> (732.1745, 47.0888) construction
  circle A4 centre (507.1745, 403.6282) radius 1.8
  circle A5 centre (527.1745, 403.6282) radius 1.8
  circle A6 centre (507.1745, 83.6282) radius 1.8
  circle A7 centre (527.1745, 83.6282) radius 1.8
  line L644 (552.1745, 373.6282) -> (912.1745, 373.6282)
  line L645 (912.1745, 373.6282) -> (912.1745, 83.6282)
  line L646 (552.1745, 83.6282) -> (552.1745, 373.6282)
  line L647 (497.1745, 228.6282) -> (967.1745, 228.6282) construction
  circle A8 centre (540.1745, 228.6282) radius 1.8
  line L648 (540.1745, 212.4782) -> (540.1745, 244.7782) construction
  line L649 (537.9245, 240.2782) -> (542.4245, 240.2782)
  line L650 (542.4245, 240.2782) -> (542.4245, 249.2782)
  line L651 (542.4245, 249.2782) -> (537.9245, 249.2782)
  line L652 (537.9245, 249.2782) -> (537.9245, 240.2782)
  line L653 (537.9245, 240.2782) -> (542.4245, 249.2782) construction
  line L654 (542.4245, 240.2782) -> (537.9245, 249.2782) construction
  line L655 (537.9245, 216.9782) -> (542.4245, 216.9782)
  line L656 (542.4245, 216.9782) -> (542.4245, 207.9782)
  line L657 (542.4245, 207.9782) -> (537.9245, 207.9782)
  line L658 (537.9245, 207.9782) -> (537.9245, 216.9782)
  line L659 (537.9245, 216.9782) -> (542.4245, 207.9782) construction
  line L660 (542.4245, 216.9782) -> (537.9245, 207.9782) construction
  circle A9 centre (924.1745, 228.6282) radius 1.8
  line L661 (924.1745, 212.4782) -> (924.1745, 244.7782) construction
  line L662 (921.9245, 240.2782) -> (926.4245, 240.2782)
  line L663 (926.4245, 240.2782) -> (926.4245, 249.2782)
  line L664 (926.4245, 249.2782) -> (921.9245, 249.2782)
  line L665 (921.9245, 249.2782) -> (921.9245, 240.2782)
  line L666 (921.9245, 240.2782) -> (926.4245, 249.2782) construction
  line L667 (926.4245, 240.2782) -> (921.9245, 249.2782) construction
  line L668 (921.9245, 216.9782) -> (926.4245, 216.9782)
  line L669 (926.4245, 216.9782) -> (926.4245, 207.9782)
  line L670 (926.4245, 207.9782) -> (921.9245, 207.9782)
  line L671 (921.9245, 207.9782) -> (921.9245, 216.9782)
  line L672 (921.9245, 216.9782) -> (926.4245, 207.9782) construction
  line L673 (926.4245, 216.9782) -> (921.9245, 207.9782) construction
  circle A10 centre (540.1745, 383.6282) radius 1.8
  line L674 (540.1745, 367.4782) -> (540.1745, 399.7782) construction
  line L675 (537.9245, 395.2782) -> (542.4245, 395.2782)
  line L676 (542.4245, 395.2782) -> (542.4245, 404.2782)
  line L677 (542.4245, 404.2782) -> (537.9245, 404.2782)
  line L678 (537.9245, 404.2782) -> (537.9245, 395.2782)
  line L679 (537.9245, 395.2782) -> (542.4245, 404.2782) construction
  line L680 (542.4245, 395.2782) -> (537.9245, 404.2782) construction
  line L681 (537.9245, 371.9782) -> (542.4245, 371.9782)
  line L682 (542.4245, 371.9782) -> (542.4245, 362.9782)
  line L683 (542.4245, 362.9782) -> (537.9245, 362.9782)
  line L684 (537.9245, 362.9782) -> (537.9245, 371.9782)
  line L685 (537.9245, 371.9782) -> (542.4245, 362.9782) construction
  line L686 (542.4245, 371.9782) -> (537.9245, 362.9782) construction
  circle A11 centre (924.1745, 383.6282) radius 1.8
  line L687 (924.1745, 367.4782) -> (924.1745, 399.7782) construction
  line L688 (921.9245, 395.2782) -> (926.4245, 395.2782)
  line L689 (926.4245, 395.2782) -> (926.4245, 404.2782)
  line L690 (926.4245, 404.2782) -> (921.9245, 404.2782)
  line L691 (921.9245, 404.2782) -> (921.9245, 395.2782)
  line L692 (921.9245, 395.2782) -> (926.4245, 404.2782) construction
  line L693 (926.4245, 395.2782) -> (921.9245, 404.2782) construction
  line L694 (921.9245, 371.9782) -> (926.4245, 371.9782)
  line L695 (926.4245, 371.9782) -> (926.4245, 362.9782)
  line L696 (926.4245, 362.9782) -> (921.9245, 362.9782)
  line L697 (921.9245, 362.9782) -> (921.9245, 371.9782)
  line L698 (921.9245, 371.9782) -> (926.4245, 362.9782) construction
  line L699 (926.4245, 371.9782) -> (921.9245, 362.9782) construction
  line L700 (524.1745, 45.6282) -> (940.1745, 45.6282)
  line L701 (940.1745, 45.6282) -> (942.1745, 43.6282)
  line L702 (524.1745, 45.6282) -> (522.1745, 43.6282)
  line L703 (497.1745, 43.6282) -> (522.1745, 43.6282)
  line L704 (942.1745, 43.6282) -> (967.1745, 43.6282)
  circle A12 centre (947.1745, 63.6282) radius 1.8
  line L705 (937.1745, 83.6282) -> (957.1745, 83.6282) construction
  line L706 (947.1745, 63.6282) -> (947.1745, 83.6282) construction
  line L707 (497.1745, 49.6282) -> (967.1745, 49.6282) construction
  circle A13 centre (917.1745, 49.6282) radius 1.8
  circle A14 centre (777.1745, 49.6282) radius 1.8
  circle A15 centre (827.1745, 49.6282) radius 1.8
  circle A16 centre (517.1745, 63.6282) radius 1.8
  circle A17 centre (547.1745, 49.6282) radius 1.8
  circle A18 centre (687.1745, 49.6282) radius 1.8
  circle A19 centre (637.1745, 49.6282) radius 1.8
  line L708 (602.1745, 83.6282) -> (602.1745, 58.6282)
  line L709 (602.1745, 58.6282) -> (612.1745, 58.6282)
  line L710 (612.1745, 58.6282) -> (612.1745, 83.6282)
  line L711 (702.1745, 83.6282) -> (727.1745, 58.6282)
  line L712 (727.1745, 58.6282) -> (737.1745, 58.6282)
  line L713 (737.1745, 58.6282) -> (762.1745, 83.6282)
  line L714 (862.1745, 83.6282) -> (862.1745, 58.6282)
  line L715 (862.1745, 58.6282) -> (852.1745, 58.6282)
  line L716 (852.1745, 58.6282) -> (852.1745, 83.6282)
  line L717 (607.1745, 58.6282) -> (607.1745, 83.6282) construction
  line L718 (602.1745, 83.6282) -> (552.1745, 83.6282)
  line L719 (702.1745, 83.6282) -> (612.1745, 83.6282)
  line L720 (912.1745, 83.6282) -> (862.1745, 83.6282)
  line L721 (852.1745, 83.6282) -> (762.1745, 83.6282)
  line L722 (926.4245, 89.2782) -> (921.9245, 89.2782)
  circle A20 centre (924.1745, 68.6282) radius 1.8
  line L723 (921.9245, 80.2782) -> (926.4245, 80.2782)
  line L724 (921.9245, 89.2782) -> (921.9245, 80.2782)
  line L725 (926.4245, 80.2782) -> (926.4245, 89.2782)
  line L726 (537.9245, 89.2782) -> (542.4245, 89.2782)
  line L727 (542.4245, 89.2782) -> (542.4245, 80.2782)
  line L728 (542.4245, 80.2782) -> (537.9245, 80.2782)
  line L729 (537.9245, 80.2782) -> (537.9245, 89.2782)
  circle A21 centre (540.1745, 68.6282) radius 1.8
  line L730 (509.6745, 49.6282) -> (525.6745, 49.6282)
  line L731 (525.6745, 49.6282) -> (525.6745, 57.6282)
  line L732 (525.6745, 57.6282) -> (509.6745, 57.6282)
  line L733 (509.6745, 57.6282) -> (509.6745, 49.6282)
  line L734 (954.6745, 49.6282) -> (938.6745, 49.6282)
  line L735 (938.6745, 49.6282) -> (938.6745, 57.6282)
  line L736 (938.6745, 57.6282) -> (954.6745, 57.6282)
  line L737 (954.6745, 57.6282) -> (954.6745, 49.6282)
  point P0 (0, 0)
  dimension "d2" = 370
  dimension "d3" = 370
  dimension "d4" = 470
  dimension "d5" = 370
  dimension "d6" = 3.5387
  dimension "d7" = 19.9743
  dimension "d8" = 320.0771
  dimension "d9" = 3.6
  dimension "d12" = 20
  dimension "d15" = 320
  dimension "d18" = 40
  dimension "d19" = 40
  dimension "d20" = 184.5341
  dimension "d21" = 260
  dimension "d22" = 290
  dimension "d23" = 360
  dimension "d24" = 290
  dimension "d25" = 32.3
  dimension "d26" = 32.3
  dimension "d27" = 9
  dimension "d28" = 6.5
  dimension "d29" = 3.6
  dimension "d30" = 3.6
  dimension "d31" = 4.5
  dimension "d32" = 9
  dimension "d33" = 32.3
  dimension "d34" = 155.0928
  dimension "d35" = 284
  dimension "d38" = 384
  dimension "d41" = 155
  dimension "d44" = 2
  dimension "d45" = 20
  dimension "d46" = 316
  dimension "d47" = 416
  dimension "d48" = 2
  dimension "d49" = 349.9119
  dimension "d50" = 450
  dimension "d51" = 10
  dimension "d53" = 20
  dimension "d61" = 4
  dimension "d62" = 50
  dimension "d63" = 140
  dimension "d64" = 90
  dimension "d65" = 4
  dimension "d66" = 3.6
  dimension "d67" = 50
  dimension "d68" = 45
  dimension "d69" = 90
  dimension "d70" = 5
  dimension "d71" = 10
  dimension "d72" = 10
  dimension "d73" = 25.0086
  dimension "d74" = 25
  dimension "d75" = 10
  dimension "d76" = 25
  dimension "d77" = 10
  dimension "d78" = 170
  dimension "d79" = 125
  dimension "d80" = 160
  dimension "d83" = 160
  dimension "d88" = 15.996
  dimension "d89" = 8
  dimension "d90" = 16
  dimension "d91" = 8
  constraints: 1476 end point, 22 centre point, 22 midpoint, 21 symmetric about line, 19 perpendicular, 14 parallel, 10 horizontal, 6 point on line, 4 coincident, 4 vertical, 3 collinear, 3 equal radius, 2 equal length, 107 other
  measures "d2" distance between parallel lines of L24 L23
  measures "d3" distance between parallel lines of L26 L2
  measures "d4" distance of L641.end L640.end
  measures "d5" distance of L640.end L640.start
  measures "d6" horizontal distance of L212.start L204.start
  measures "d7" distance of L194.start L171.end
  measures "d8" distance of L261.end L205.end
  measures "d9" diameter of A0
  measures "d12" distance of A0.centre A1.centre
  measures "d15" distance of A0.centre L705.end
  measures "d18" distance between parallel lines of L2 L12
  measures "d19" distance between parallel lines of L25 L16
  measures "d20" distance from line of L2 L122.end
  measures "d21" distance between parallel lines of L10 L14
  measures "d22" distance from line of L16.end L12
  measures "d23" distance of L644.start L644.end
  measures "d24" distance of L646.start L644.start
  measures "d25" distance between parallel lines of L97 L93
  measures "d26" distance between parallel lines of L89 L85
  measures "d27" distance of L95.end L96.end
  measures "d28" distance of L96.end L94.start
  measures "d29" distance of L133.end L122.start
  measures "d30" diameter of A8
  measures "d31" distance of L651.end L650.end
  measures "d32" distance of L650.end L649.end
  measures "d33" distance of L648.start L648.end
  measures "d34" distance between parallel lines of L85 L93
  measures "d35" distance between parallel lines of L106 L86
  measures "d38" distance of L650.end L664.start
  measures "d41" distance of L650.end L677.start
  measures "d44" distance between parallel lines of L6 L26
  measures "d45" distance of L7.end L0.start
  measures "d46" distance of L5.end L7.start
  measures "d47" distance of L700.start L700.end
  measures "d48" distance between parallel lines of L700 L703
  measures "d49" distance of L212.start L454.start
  measures "d50" distance of A0.centre A4.centre
  measures "d51" distance from line of L641 A5.centre
  measures "d53" distance of L706.start L706.end
  measures "d61" distance from line of L590.start L6
  measures "d62" distance from line of L596.start L24
  measures "d63" distance from line of L559.end L24
  measures "d64" distance of L547.end L572.start
  measures "d65" distance between parallel lines of L700 L707
  measures "d66" diameter of A13
  measures "d67" distance from line of L640 A13.centre
  measures "d68" distance from line of L643 A14.centre
  measures "d69" distance of A15.centre A13.centre
  measures "d70" horizontal distance of L11.end L10.end
  measures "d71" distance between parallel lines of L632 L619
  measures "d72" distance between parallel lines of L710 L708
  measures "d73" distance from line of L20 L608.end
  measures "d74" distance of L708.start L708.end
  measures "d75" distance of L17.start L18.start
  measures "d76" distance between parallel lines of L17 L20
  measures "d77" distance of L711.end L712.end
  measures "d78" distance between parallel lines of L632 L615
  measures "d79" distance between parallel lines of L643 L717
  measures "d80" distance between parallel lines of L111 L119
  measures "d83" distance of L664.start L722.start
  measures "d88" distance of L51.start L28.start
  measures "d89" distance from line of L30.end L55
  measures "d90" distance of L732.end L731.end
  measures "d91" distance of L731.end L730.end
extrude "Extrusion1" add sketch "Sketch1" along normal blind 4 contours L704 L701 L700 L702 L703 L642 L641 L640
chamfer "Chamfer1" distance 5 angle 45 8 edges at (967.1745, 43.6282, 2) (967.1745, 413.6282, 2) (497.1745, 413.6282, 2) (497.1745, 43.6282, 2) (912.1745, 83.6282, 2) (912.1745, 373.6282, 2) (552.1745, 373.6282, 2) (552.1745, 83.6282, 2)
fillet "Fillet1" radius 5 4 edges at (602.1745, 58.6282, 2) (612.1745, 58.6282, 2) (862.1745, 58.6282, 2) (852.1745, 58.6282, 2)
fillet "Fillet2" radius 4 8 edges at (938.6745, 49.6282, 2) (938.6745, 57.6282, 2) (954.6745, 49.6282, 2) (954.6745, 57.6282, 2) (509.6745, 49.6282, 2) (509.6745, 57.6282, 2) (525.6745, 57.6282, 2) (525.6745, 49.6282, 2)
body "Solid1"
